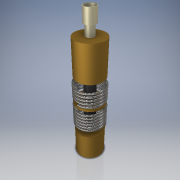
# Autodesk Inventor part: minifridge
Saved by Autodesk Inventor 2018 (Build 220112000, 112)
## iProperties
Created: 2019-03-15
Part Number: minifridge
Material: Brass, Soft Yellow
Document SubType Name: Modeling
Designer: Admin
Density: 8.47 g/cm^3
Appearance: Sky Blue Dark
Author: Admin
Autodesk Inventor part; units mm, degrees
ref_plane "YZ Plane" through (0, 0, 0) normal (1, 0, 0) x (0, 1, 0)
ref_plane "XZ Plane" through (0, 0, 0) normal (0, 1, 0) x (-1, 0, 0)
ref_plane "XY Plane" through (0, 0, 0) normal (0, 0, 1) x (1, 0, 0)
sketch "Sketch3" plane through (0, 0, 0) normal (0, 1, 0) x (-1, 0, 0)
  circle A0 centre (0, 0) radius 5.588
  circle A1 centre (0, 0) radius 6.35
  dimension "d6" = 11.176
  dimension "d7" = 12.7
  constraints: 2 centre point, 2 coincident
  measures "d6" diameter of A0
  measures "d7" diameter of A1
extrude "Extrusion3" add sketch "Sketch3" along normal blind 11.176
sketch "Sketch4" plane through (0, 0, 0) normal (0, -1, 0) x (1, 0, 0)
  circle A0 centre (0, 0) radius 3.81
  circle A1 centre (0, 0) radius 6.35
  circle A2 centre (0, 0) radius 6.35 projected
  dimension "d10" = 7.62
  constraints: 2 centre point, 2 coincident, 1 concentric
  measures "d10" diameter of A0
extrude "Extrusion4" add sketch "Sketch4" along normal blind 2.54
sketch "Sketch5" plane through (0, -2.54, 0) normal (0, -1, 0) x (1, 0, 0)
  circle A0 centre (0, 0) radius 3.81
  circle A1 centre (0, 0) radius 4.572
  circle A2 centre (0, 0) radius 3.81 projected
  dimension "d13" = 0.762
  constraints: 2 centre point, 2 coincident, 1 concentric
  measures "d13" radial gap between concentric circles of A0 A1
extrude "Extrusion5" add sketch "Sketch5" along normal blind 11.176
sketch "Sketch6" plane through (0, -13.716, 0) normal (0, -1, 0) x (1, 0, 0)
  circle A0 centre (0, 0) radius 15.875
  dimension "d16" = 31.75
  constraints: 1 centre point, 1 coincident
  measures "d16" diameter of A0
extrude "Extrusion6" add sketch "Sketch6" along normal blind 38.1
sketch "Sketch7" plane through (0, -51.816, 0) normal (0, -1, 0) x (1, 0, 0)
  circle A0 centre (0, 0) radius 6.35
  dimension "d19" = 12.7
  constraints: 1 centre point, 1 coincident
  measures "d19" diameter of A0
extrude "Extrusion7" add sketch "Sketch7" along normal blind 63.5
sketch "Sketch8" plane through (0, 0, 0) normal (1, 0, 0) x (0, 1, 0)
  line L0 (-115.316, 6.35) -> (-115.316, -6.35) projected
  circle A0 centre (-83.566, 15.875) radius 1.27
  line L1 (-51.816, 15.875) -> (-51.816, -15.875) projected
  line L2 (-51.816, 0) -> (-83.566, 0)
  line L3 (-83.566, 0) -> (-83.566, 15.875)
  point P0 (0, 0)
  dimension "d23" = 2.54
  dimension "d32" = 15.875
  dimension "d33" = 31.75
  constraints: 4 end point, 1 centre point, 1 coincident, 1 horizontal, 1 midpoint, 1 perpendicular
  measures "d23" diameter of A0
  measures "d32" distance of L2.end L3.end
  measures "d33" distance of L2.start L2.end
coil "Coil1" sketch "Sketch8" operation add axis through (0, -10, 0) along (0, -1, 0) pitch 3.81 turns 6.666667 hand right
sketch "Sketch9" plane through (0, -115.316, 0) normal (0, -1, 0) x (1, 0, 0)
  circle A0 centre (0, 0) radius 3.81 projected
  circle A1 centre (0, 0) radius 15.875
  dimension "d34" = 31.75
  constraints: 1 centre point, 1 coincident
  measures "d34" diameter of A1
extrude "Extrusion8" add sketch "Sketch9" along normal blind 31.75 contours A0 | A1
sketch "Sketch10" plane through (0, 57.658, -0.635) normal (1, 0, 0) x (0, 1, 0)
  circle A0 centre (-115.824, 16.51) radius 1.27
  line L0 (-109.474, 17.145) -> (-109.474, -15.875)
  line L1 (-109.474, 0.635) -> (-115.824, 0.635)
  line L2 (-115.824, 0.635) -> (-115.824, 16.51)
  line L3 (-109.474, 16.51) -> (-109.474, -15.24) projected
  line L4 (-71.374, -3.175) -> (-71.374, 4.445) projected
  line L5 (-71.374, 0.635) -> (-109.474, 0.635)
  point P0 (0, 0)
  dimension "d47" = 2.54
  dimension "d45" = 15.875
  dimension "d48" = 6.35
  constraints: 8 end point, 4 midpoint, 2 horizontal, 2 perpendicular, 1 centre point, 1 coincident, 1 collinear
  measures "d47" diameter of A0
  measures "d45" distance of L1.end L2.end
  measures "d48" distance between parallel lines of L2 L0
coil "Coil2" sketch "Sketch10" operation add axis through (0, -13.716, 0) along (0, -1, 0) pitch 3.81 turns 5 hand right
sketch "Sketch11" plane through (0, 0, 0) normal (1, 0, 0) x (0, 1, 0)
  line L0 (0, 0) -> (-78.74, 0)
  line L1 (-78.74, 0) -> (-81.28, 0)
  line L2 (-81.28, 0) -> (-81.28, -16.51)
  line L3 (-81.28, -16.51) -> (-78.74, -16.51)
  line L4 (-78.74, -16.51) -> (-78.74, 0)
  dimension "d49" = 2.54
  dimension "d50" = 16.51
  dimension "d52" = 78.74
  constraints: 10 end point, 2 horizontal, 2 parallel, 1 perpendicular
  measures "d49" distance of L3.end L2.end
  measures "d50" distance of L2.end L1.end
  measures "d52" distance of L0.start L0.end
revolve "Revolution1" add sketch "Sketch11" angle 360 about axis through (0, 0, 0) along (0, -1, 0)
body "Solid2"
